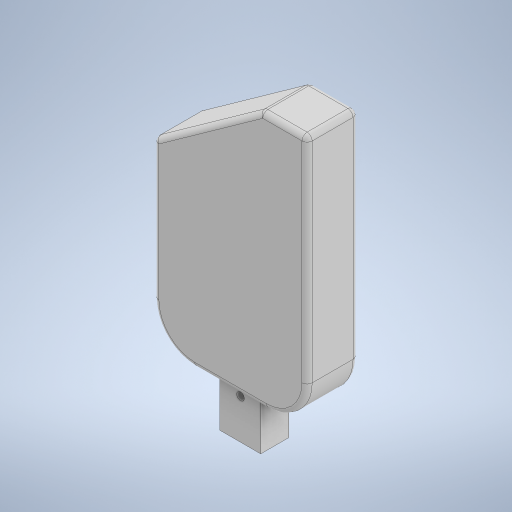
# Autodesk Inventor part: Part1
Saved by Autodesk Inventor 2023.5 (Build 275446020, 446B)
## iProperties
Created: 2025-04-21
Part Number: Part1
Material: Generic
Document SubType Name: Modeling
Designer: Lucky Sah
Density: 1 g/cm^3
Appearance: Default
Author: Lucky Sah
Autodesk Inventor part; units mm, degrees
ref_plane "YZ Plane" through (0, 0, 0) normal (1, 0, 0) x (0, 1, 0)
ref_plane "XZ Plane" through (0, 0, 0) normal (0, 1, 0) x (-1, 0, 0)
ref_plane "XY Plane" through (0, 0, 0) normal (0, 0, 1) x (1, 0, 0)
sketch "Sketch1" plane through (0, 0, 0) normal (0, 0, 1) x (1, 0, 0)
  line L0 (8, 0) -> (22, 0)
  line L1 (30, 8) -> (30, 50)
  line L2 (30, 50) -> (0, 50)
  line L3 (0, 50) -> (0, 8)
  line L4 (0, 50) -> (0, 35)
  line L5 (30, 50) -> (21, 50)
  line L6 (21, 50) -> (0, 35)
  arc A0 (0, 8) -> (8, 0) centre (8, 8) ccw
  arc A1 (22, 0) -> (30, 8) centre (22, 8) ccw
  point P0 (0, 0)
  point P1 (30, 0)
  dimension "d0" = 30
  dimension "d1" = 50
  dimension "d2" = 15
  dimension "d3" = 9
  dimension "d4" = 8
  constraints: 14 end point, 6 point on line, 4 point on circle, 4 tangent, 2 centre point, 2 parallel, 1 equal radius, 1 horizontal, 1 perpendicular
  measures "d0" distance of L2.end L1.end
  measures "d1" distance of L1.end point (30, 0)
  measures "d2" distance of L2.end L4.end
  measures "d3" distance of L1.end L5.end
  measures "d4" radius of A0
extrude "Extrusion1" add sketch "Sketch1" along normal blind 10 contours A0 L3 L6 L2 L1 A1 L0
fillet "Fillet1" radius 1 17 edges at (2.3431, 2.3431, 10) (15, 0, 10) (27.6569, 2.3431, 10) (30, 29, 10) (0, 21.5, 10) (10.5, 42.5, 10) (25.5, 50, 10) (25.5, 50, 0) (10.5, 42.5, 0) (2.3431, 2.3431, 0) (15, 0, 0) (27.6569, 2.3431, 0) (30, 29, 0) (0, 21.5, 0) (0, 35, 5) (21, 50, 5) (30, 50, 5)
sketch "Sketch2" plane through (8, 0, 9) normal (0, -1, 0) x (1, 0, 0)
  line L0 (4.5, -4.925) -> (9.5, -4.925)
  line L1 (9.5, -4.925) -> (9.5, -2.425)
  line L2 (9.5, -2.425) -> (4.5, -2.425)
  line L3 (4.5, -2.425) -> (4.5, -4.925)
  line L4 (22, -8) -> (22, 0) projected
  line L5 (-8, -8) -> (-8, 0) projected
  line L6 (0, -9) -> (14, -9) projected
  line L7 (14, 1) -> (0, 1) projected
  line L8 (11, -6.425) -> (3, -6.425)
  line L9 (3, -6.425) -> (3, -0.925)
  line L10 (3, -0.925) -> (11, -0.925)
  line L11 (11, -0.925) -> (11, -6.425)
  point P0 (-8, -9)
  dimension "d8" = 5
  dimension "d9" = 2.5
  dimension "d10" = 30
  dimension "d11" = 12.5
  dimension "d12" = 10
  dimension "d13" = 3.425
  dimension "d14" = 1.5
  constraints: 16 end point, 4 parallel, 2 perpendicular, 1 horizontal, 3 other
  measures "d8" distance of L2.end L1.end
  measures "d9" distance of L1.end L0.end
  measures "d10" distance between parallel lines of L4 L5
  measures "d11" distance between parallel lines of L5 L3
  measures "d12" distance between parallel lines of L6 L7
  measures "d13" distance between parallel lines of L7 L2
  measures "d14" distance between parallel lines of L0 L8
extrude "Extrusion2" add sketch "Sketch2" along normal blind 10
sketch "Sketch3" plane through (11, 0, 8.075) normal (0, 0, 1) x (1, 0, 0)
  circle A0 centre (4.0603, -2.2) radius 0.75
  line L0 (8, -10) -> (0, -10) projected
  point P0 (-11, 0)
  dimension "d17" = 1.5
  dimension "d18" = 7.8
  constraints: 1 centre point
  measures "d17" diameter of A0
  measures "d18" distance from line of L0 A0.centre
extrude "Extrusion3" cut sketch "Sketch3" against normal up to surface (5.5 mm away)
body "Solid1"
